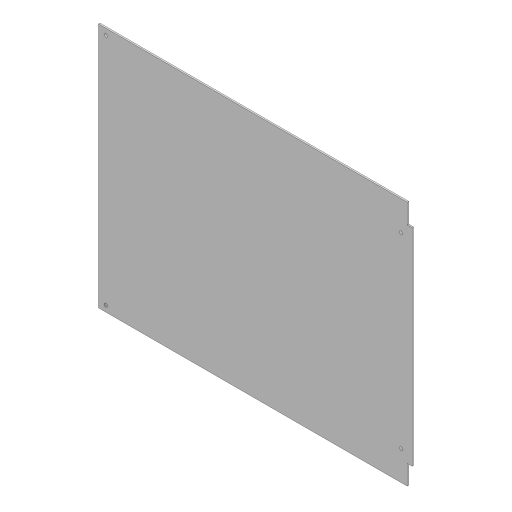
# Autodesk Inventor part: right_wall
Saved by Autodesk Inventor 2023 (Build 270158000, 158)
## iProperties
Created: 2024-06-07
Part Number: right_wall
Material: Generic
Document SubType Name: Modeling
Designer: nvladi
Density: 1 g/cm^3
Appearance: Default
Author: nvladi
Autodesk Inventor part; units mm, degrees
ref_plane "YZ Plane" through (0, 0, 0) normal (1, 0, 0) x (0, 1, 0)
ref_plane "XZ Plane" through (0, 0, 0) normal (0, 1, 0) x (-1, 0, 0)
ref_plane "XY Plane" through (0, 0, 0) normal (0, 0, 1) x (1, 0, 0)
sketch "Sketch1" plane through (0, 0, 0) normal (0, 0, 1) x (1, 0, 0)
  line L0 (638, 0) -> (0, 0)
  line L1 (0, 0) -> (0, 500)
  line L2 (0, 500) -> (638, 500)
  line L3 (638, 500) -> (638, 0)
  line L4 (615.5, 493.1922) -> (615.5, 30.4656) construction
  line L5 (15.5, 487.5) -> (15.5, 12.5) construction
  line L6 (638, 500) -> (615.5, 500)
  line L7 (638, 460) -> (638, 500)
  line L8 (638, 0) -> (615.5, 0)
  line L9 (638, 40) -> (638, 0)
  line L10 (638, 500) -> (628, 500)
  line L11 (628, 500) -> (628, 460)
  line L12 (628, 460) -> (638, 460)
  line L13 (638, 460) -> (638, 500)
  line L14 (638, 0) -> (628, 0)
  line L15 (628, 0) -> (628, 40)
  line L16 (628, 40) -> (638, 40)
  line L17 (638, 40) -> (638, 0)
  point P0 (615.5, 60)
  point P1 (615.5, 440)
  point P2 (615.5, 40)
  dimension "d2" = 638
  dimension "d3" = 500
  dimension "d10" = 22.5
  dimension "d11" = 15.5
  dimension "d12" = 12.5
  dimension "d13" = 12.5
  dimension "d14" = 60
  dimension "d15" = 60
  dimension "d29" = 10
  constraints: 36 end point, 7 parallel, 5 horizontal, 3 perpendicular, 3 point on line, 1 vertical
  measures "d2" distance of L1.end L2.end
  measures "d3" distance of L0.end L1.end
  measures "d10" distance between parallel lines of L3 L4
  measures "d11" distance between parallel lines of L5 L1
  measures "d12" distance from line of L5.start L2
  measures "d13" distance from line of L0 L5.end
  measures "d14" distance from line of L0 point (615.5, 60)
  measures "d15" distance from line of L2 point (615.5, 440)
  measures "d29" distance of L12.end L11.end
extrude "Extrusion1" add sketch "Sketch1" along normal blind 3
hole "Hole1" at (615.5, 60, 0) at (615.5, 440, 0) at (15.5, 487.5, 0) at (15.5, 12.5, 0) direction (0, 0, 1) diameter 6.4 end through all
extrude "Extrusion3" cut sketch "Sketch1" along normal through all contours L0 L15 L16 L3 | L12 L11 L2 L3
body "Solid1"
